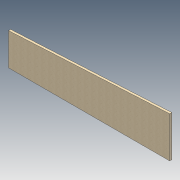
# Autodesk Inventor part: GE-12103-01
Saved by Autodesk Inventor 2012 (Build 160160000, 160)
## iProperties
Created: 2011-11-27
Part Number: GE-12103-01
Document SubType Name: Modeling
Designer: dfoster
Density: 1 g/cm^3
Description: Side, Plywood
Material: Default
Title: Side, Plywood
Author: dfoster
Autodesk Inventor part; units mm, degrees
ref_plane "YZ Plane" through (0, 0, 0) normal (1, 0, 0) x (0, 1, 0)
ref_plane "XZ Plane" through (0, 0, 0) normal (0, 1, 0) x (-1, 0, 0)
ref_plane "XY Plane" through (0, 0, 0) normal (0, 0, 1) x (1, 0, 0)
sketch "Sketch1" plane through (0, 0, 0) normal (0, 0, 1) x (1, 0, 0)
  line L0 (0, 0) -> (0, 190.5)
  line L1 (0, 190.5) -> (952.5, 241.3)
  line L2 (952.5, 241.3) -> (952.5, 0)
  line L3 (952.5, 0) -> (0, 0)
  dimension "d0" = 952.5
  dimension "d5" = 190.5
  dimension "d9" = 241.3
  constraints: 8 end point, 2 vertical, 1 horizontal
  measures "d0" distance of L2.end L0.start
  measures "d5" distance of L0.start L0.end
  measures "d9" distance of L1.end L2.end
extrude "Extrusion1" add sketch "Sketch1" along normal blind 12.7
body "Solid1"
